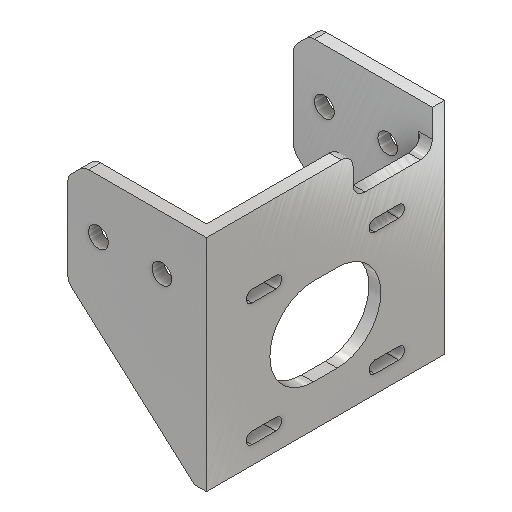
# Autodesk Inventor part: CNCM_ALU_Y_Axis_Nema_17_Mount
Saved by Autodesk Inventor 2026.1 (Build 301233000, 233)
## iProperties
Created: 2016-03-27
Part Number: CNCM_ALU_Y_Axis_Nema_17_Mount
Material: Ogólny
Document SubType Name: Modeling
Designer: Andrzej
Density: 1 g/cm^3
Appearance: Obrobione — aluminium
Mass: 15.9975 g
Surface Area: 120.32 cm^2
Volume: 15.9975 cm^3
Author: Andrzej
Autodesk Inventor part; units mm, degrees
ref_plane "YZ Plane" through (0, 0, 0) normal (1, 0, 0) x (0, 1, 0)
ref_plane "XZ Plane" through (0, 0, 0) normal (0, 1, 0) x (-1, 0, 0)
ref_plane "XY Plane" through (0, 0, 0) normal (0, 0, 1) x (1, 0, 0)
sketch "Szkic1" plane through (0, 0, 0) normal (0, 0, 1) x (1, 0, 0)
  line L0 (-24.1556, -3.6171) -> (-24.1556, -6.6171)
  line L1 (-24.1556, -6.6171) -> (10.8444, -6.6171)
  line L2 (10.8444, -6.6171) -> (10.8444, 53.3829)
  line L3 (7.8444, 50.3829) -> (7.8444, -3.6171)
  line L4 (7.8444, -3.6171) -> (-24.1556, -3.6171)
  line L5 (-24.1556, 53.3829) -> (-24.1556, 50.3829)
  line L6 (-24.1556, 50.3829) -> (7.8444, 50.3829)
  line L7 (-24.1556, 53.3829) -> (10.8444, 53.3829)
  point P0 (0, 0)
  dimension "d2" = 60
  dimension "d87" = 3
  dimension "d89" = 3
  dimension "d90" = 3
  dimension "d123" = 35
  dimension "d124" = 35
  constraints: 16 end point, 4 perpendicular, 1 horizontal, 1 vertical
  measures "d2" distance of L1.end L2.end
  measures "d87" distance of L5.start L5.end
  measures "d89" distance between parallel lines of L2 L3
  measures "d90" distance between parallel lines of L4 L1
  measures "d123" distance between parallel lines of L2 L5
  measures "d124" distance between parallel lines of L0 L2
extrude "Wyciągnięcie proste1" add sketch "Szkic1" along normal blind 55.5
fillet "Zaokrąglenie1" radius 0.5 2 edges at (7.8444, -3.6171, 27.75) (7.8444, 50.3829, 27.75)
sketch "Szkic9" plane through (7.8444, -3.1171, 0) normal (-1, 0, 0) x (0, 0, 1)
  line L0 (42.5, 5.5) -> (0.5, 5.5)
  line L1 (0.5, 5.5) -> (0.5, 47.5)
  line L2 (0.5, 47.5) -> (42.5, 47.5)
  line L3 (42.5, 47.5) -> (42.5, 5.5)
  line L4 (0, 53) -> (55.5, 53) projected
  line L5 (0, 53) -> (0, 0) projected
  line L6 (55.5, 0) -> (0, 0) projected
  line L7 (55.5, 53) -> (55.5, 0) projected
  line L8 (37, 14) -> (37, 8) construction
  line L9 (35.5, 14) -> (35.5, 8)
  line L10 (38.5, 8) -> (38.5, 14)
  arc A0 (38.5, 14) -> (35.5, 14) centre (37, 14) ccw
  arc A1 (35.5, 8) -> (38.5, 8) centre (37, 8) ccw
  line L11 (37, 45) -> (37, 39) construction
  line L12 (35.5, 45) -> (35.5, 39)
  line L13 (38.5, 39) -> (38.5, 45)
  arc A2 (38.5, 45) -> (35.5, 45) centre (37, 45) ccw
  arc A3 (35.5, 39) -> (38.5, 39) centre (37, 39) ccw
  line L14 (6, 14) -> (6, 8) construction
  line L15 (4.5, 14) -> (4.5, 8)
  line L16 (7.5, 8) -> (7.5, 14)
  arc A4 (7.5, 14) -> (4.5, 14) centre (6, 14) ccw
  arc A5 (4.5, 8) -> (7.5, 8) centre (6, 8) ccw
  line L17 (6, 45) -> (6, 39) construction
  line L18 (4.5, 45) -> (4.5, 39)
  line L19 (7.5, 39) -> (7.5, 45)
  arc A6 (7.5, 45) -> (4.5, 45) centre (6, 45) ccw
  arc A7 (4.5, 39) -> (7.5, 39) centre (6, 39) ccw
  line L20 (21.5, 29.5) -> (21.5, 23.5) construction
  line L21 (10.5, 29.5) -> (10.5, 23.5)
  line L22 (32.5, 23.5) -> (32.5, 29.5)
  arc A8 (32.5, 29.5) -> (10.5, 29.5) centre (21.5, 29.5) ccw
  arc A9 (10.5, 23.5) -> (32.5, 23.5) centre (21.5, 23.5) ccw
  point P0 (0, 3.1171)
  point P1 (37, 11)
  point P2 (6, 11)
  point P3 (37, 42)
  point P4 (6, 42)
  point P5 (21.5, 26.5)
  dimension "d128" = 42
  dimension "d129" = 42
  dimension "d130" = 5.5
  dimension "d131" = 0.5
  dimension "d132" = 53
  dimension "d133" = 5.5
  dimension "d134" = 5.5
  dimension "d135" = 5.5
  dimension "d136" = 5.5
  dimension "d137" = 5.5
  dimension "d138" = 5.5
  dimension "d139" = 5.5
  dimension "d140" = 5.5
  dimension "d141" = 21
  dimension "d142" = 21
  dimension "d143" = 3
  dimension "d144" = 3
  dimension "d145" = 3
  dimension "d146" = 3
  dimension "d147" = 3
  dimension "d148" = 3
  dimension "d149" = 3
  dimension "d150" = 3
  dimension "d151" = 3
  dimension "d152" = 22
  constraints: 48 end point, 20 point on circle, 20 tangent, 10 centre point, 8 parallel, 5 midpoint, 2 point on line, 2 vertical, 1 horizontal, 1 perpendicular
  measures "d128" distance of L1.end L2.end
  measures "d129" distance of L0.end L1.end
  measures "d130" distance between parallel lines of L0 L6
  measures "d131" distance between parallel lines of L5 L1
  measures "d132" distance between parallel lines of L6 L4
  measures "d133" distance from line of L3 point (37, 11)
  measures "d134" distance from line of L0 point (37, 11)
  measures "d135" distance from line of L0 point (6, 11)
  measures "d136" distance from line of L1 point (6, 11)
  measures "d137" distance from line of L3 point (37, 42)
  measures "d138" distance from line of L2 point (37, 42)
  measures "d139" distance from line of L2 point (6, 42)
  measures "d140" distance from line of L1 point (6, 42)
  measures "d141" distance from line of L0 point (21.5, 26.5)
  measures "d142" distance from line of L3 point (21.5, 26.5)
  measures "d143" distance of point (37, 11) L8.end
  measures "d144" diameter of A1
  measures "d145" distance of point (37, 42) L11.end
  measures "d146" diameter of A3
  measures "d147" distance of point (6, 11) L14.end
  measures "d148" diameter of A5
  measures "d149" distance of point (6, 42) L17.end
  measures "d150" diameter of A7
  measures "d151" distance of point (21.5, 26.5) L20.end
  measures "d152" diameter of A9
extrude "Wyciągnięcie proste4" cut sketch "Szkic9" against normal blind 3 contours A0 L10 A1 L9 | A2 L13 A3 L12 | A4 L16 A5 L15 | A6 L19 A7 L18 | A8 L22 A9 L21
sketch "Szkic10" plane through (-24.1556, -6.6171, 0) normal (0, -1, 0) x (1, 0, 0)
  line L0 (0, 0) -> (35, 0) projected
  line L1 (35, 0) -> (35, 55.5) projected
  line L2 (0, 55.5) -> (35, 55.5) projected
  line L3 (0, 0) -> (0, 55.5) projected
  line L4 (32, 55.5) -> (32, 0) projected
  line L5 (0, 28.5) -> (32, 28.5)
  line L6 (32, 10.5) -> (32, 32.5) projected
  line L7 (0, 28.5) -> (32, 0)
  point P0 (24.1556, 0)
  dimension "d155" = 28.5
  constraints: 4 end point, 2 point on line, 1 perpendicular
  measures "d155" distance between parallel lines of L0 L5
extrude "Wyciągnięcie proste5" cut sketch "Szkic10" against normal up to surface (60 mm away) contours L3 L7 L0
sketch "Szkic11" plane through (-24.1556, -6.6171, 55.5) normal (0, -1, 0) x (1, 0, 0)
  line L0 (0, -27) -> (32, -55.5) projected
  line L1 (32, -55.5) -> (35, -55.5) projected
  line L2 (35, -55.5) -> (35, 0) projected
  line L3 (0, 0) -> (35, 0) projected
  line L4 (0, -27) -> (0, 0) projected
  line L5 (31.5, -55.0547) -> (31.5, 0) projected
  line L6 (32, 0) -> (32, -55.5) projected
  point P0 (24.1556, -55.5)
  point P1 (7.75, -13.5)
  point P2 (23.75, -13.5)
  dimension "d158" = 13.5
  dimension "d159" = 13.5
  dimension "d160" = 16
  dimension "d161" = 31.5
  dimension "d162" = 7.75
  measures "d158" distance from line of point (7.75, -13.5) L3
  measures "d159" distance from line of L3 point (23.75, -13.5)
  measures "d160" distance of point (7.75, -13.5) point (23.75, -13.5)
  measures "d161" distance between parallel lines of L4 L5
  measures "d162" distance from line of L5 point (23.75, -13.5)
hole "Otwór7" at (-16.4056, -6.6171, 42) at (-0.4056, -6.6171, 42) direction (0, 1, 0) diameter 5 end through all
chamfer "Faza5" distance 4 angle 45 2 edges at (-24.1556, -5.1171, 55.5) (-24.1556, 51.8829, 55.5)
fillet "Zaokrąglenie6" radius 3 6 edges at (-24.1556, -5.1171, 28.5) (-24.1556, 51.8829, 28.5) (-24.1556, 51.8829, 51.5) (-20.1556, 51.8829, 55.5) (-24.1556, -5.1171, 51.5) (-20.1556, -5.1171, 55.5)
sketch "Szkic12" plane through (10.8444, -6.6171, 0) normal (1, 0, 0) x (0, 0, -1)
  line L0 (-55.5, 57) -> (-0.4453, 57) projected
  arc A0 (-7.5, 42.5) -> (-4.5, 42.5) centre (-6, 42.5) ccw projected
  line L1 (-7.5, 42.5) -> (-7.5, 48.5) projected
  arc A1 (-4.5, 48.5) -> (-7.5, 48.5) centre (-6, 48.5) ccw projected
  line L2 (-4.5, 48.5) -> (-4.5, 42.5) projected
  arc A2 (-38.5, 42.5) -> (-35.5, 42.5) centre (-37, 42.5) ccw projected
  line L3 (-38.5, 42.5) -> (-38.5, 48.5) projected
  arc A3 (-35.5, 48.5) -> (-38.5, 48.5) centre (-37, 48.5) ccw projected
  line L4 (-35.5, 48.5) -> (-35.5, 42.5) projected
  arc A4 (-38.5, 11.5) -> (-35.5, 11.5) centre (-37, 11.5) ccw projected
  line L5 (-38.5, 11.5) -> (-38.5, 17.5) projected
  arc A5 (-35.5, 17.5) -> (-38.5, 17.5) centre (-37, 17.5) ccw projected
  line L6 (-35.5, 17.5) -> (-35.5, 11.5) projected
  arc A6 (-7.5, 11.5) -> (-4.5, 11.5) centre (-6, 11.5) ccw projected
  line L7 (-7.5, 11.5) -> (-7.5, 17.5) projected
  arc A7 (-4.5, 17.5) -> (-7.5, 17.5) centre (-6, 17.5) ccw projected
  line L8 (-4.5, 17.5) -> (-4.5, 11.5) projected
  arc A8 (-32.5, 27) -> (-10.5, 27) centre (-21.5, 27) ccw projected
  line L9 (-32.5, 27) -> (-32.5, 33) projected
  arc A9 (-10.5, 33) -> (-32.5, 33) centre (-21.5, 33) ccw projected
  line L10 (-10.5, 33) -> (-10.5, 27) projected
  line L11 (0, 0) -> (0, 60) projected
  line L12 (0, 60) -> (-55.5, 60) projected
  line L13 (-55.5, 0) -> (-55.5, 60) projected
  line L14 (0, 0) -> (-55.5, 0) projected
  line L15 (-0.4453, 3) -> (-55.5, 3) projected
  line L16 (-55.5, 57) -> (-45.5, 57)
  line L17 (-45.5, 57) -> (-45.5, 37)
  line L18 (-45.5, 37) -> (-55.5, 37)
  line L19 (-55.5, 37) -> (-55.5, 57)
  point P0 (0, 6.6171)
  dimension "d174" = 20
  dimension "d175" = 10
  constraints: 8 end point, 2 parallel, 1 horizontal, 1 perpendicular
  measures "d174" distance of L16.end L17.end
  measures "d175" distance of L17.end L18.end
extrude "Wyciągnięcie proste6" cut sketch "Szkic12" against normal through all contours L0 L17 L18 L13
fillet "Zaokrąglenie7" radius 3 3 edges at (9.0944, 50.3829, 45.5) (9.3444, 30.3829, 45.5) (9.3444, 30.3829, 55.5)
equation "\"d124\" = d123"
equation "\"d130\" = -0.5 * d129 + 0.5 * d132"
equation "\"d134\" = d133"
equation "\"d135\" = d133"
equation "\"d136\" = d133"
equation "\"d137\" = d133"
equation "\"d138\" = d133"
equation "\"d139\" = d133"
equation "\"d140\" = d133"
equation "\"d141\" = 0.5 * d129"
equation "\"d142\" = d141"
equation "\"d159\" = d158"
equation "\"d162\" = -0.5 * d160 + 0.5 * d161"
